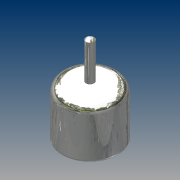
# Autodesk Inventor part: MotorTop
Saved by Autodesk Inventor 2011 SP1 (Build 150282100, 282)
## iProperties
Created: 2011-07-19
Part Number: MotorTop
Document SubType Name: Modeling
Designer: Nathan
Density: 1 g/cm^3
Author: Nathan
Autodesk Inventor part; units mm, degrees
ref_plane "YZ Plane" through (0, 0, 0) normal (1, 0, 0) x (0, 1, 0)
ref_plane "XZ Plane" through (0, 0, 0) normal (0, 1, 0) x (-1, 0, 0)
ref_plane "XY Plane" through (0, 0, 0) normal (0, 0, 1) x (1, 0, 0)
sketch "Sketch1" plane through (0, 0, 0) normal (0, 0, 1) x (1, 0, 0)
  line L0 (0, 0) -> (-13.97, 0)
  line L1 (-13.97, 0) -> (-13.97, 25.4)
  line L2 (0, 43.18) -> (0, 0)
  line L3 (-13.97, 25.4) -> (-2, 25.4)
  line L4 (-2, 25.4) -> (-2, 43.18)
  line L5 (-2, 43.18) -> (0, 43.18)
  dimension "d16" = 25.4
  dimension "d17" = 13.97
  dimension "d18" = 2
  dimension "d19" = 17.78
  constraints: 12 end point, 3 perpendicular, 2 parallel, 1 horizontal, 1 other
  measures "d16" distance of L0.end L1.end
  measures "d17" distance between parallel lines of L2 L1
  measures "d18" distance between parallel lines of L2 L4
  measures "d19" distance of L3.end L4.end
revolve "Revolution1" add sketch "Sketch1" angle 360 about axis through (0, 43.18, 0) along (0, -1, 0)
fillet "Fillet1" radius 4.7625 1 edges at (13.97, 25.4, 0)
fillet "Fillet2" radius 1.5875 1 edges at (13.97, 0, 0)
body "Solid1"
